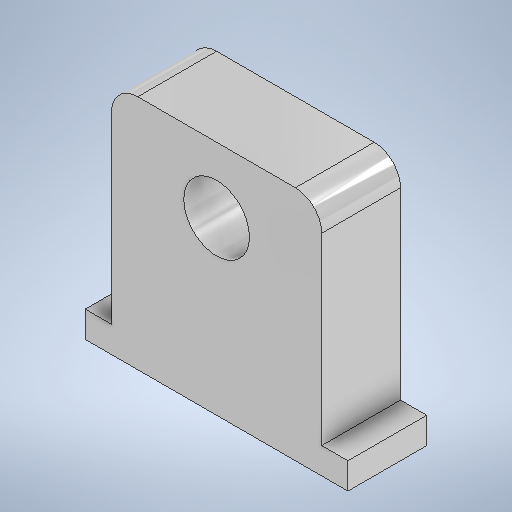
# Autodesk Inventor part: Base
Saved by Autodesk Inventor 2025 (Build 290162000, 162)
## iProperties
Created: 2023-05-05
Part Number: Base
Material: Aluminio 6061
Document SubType Name: Modeling
Designer: Miguel Ángel
Density: 2.69921 g/cm^3
Appearance: Aluminio - Oscuro
Mass: 556 g
Surface Area: 272.311 cm^2
Volume: 205.986 cm^3
Author: Miguel Ángel
Autodesk Inventor part; units mm, degrees
ref_plane "YZ Plane" through (0, 0, 0) normal (1, 0, 0) x (0, 1, 0)
ref_plane "XZ Plane" through (0, 0, 0) normal (0, 1, 0) x (-1, 0, 0)
ref_plane "XY Plane" through (0, 0, 0) normal (0, 0, 1) x (1, 0, 0)
sketch "Boceto1" plane through (0, 0, 0) normal (0, 0, 1) x (1, 0, 0)
  circle A0 centre (0, 0) radius 12.5
  line L0 (0, 25) -> (30, 25)
  line L1 (40, 15) -> (40, -55)
  line L2 (40, -55) -> (50, -55)
  line L3 (50, -55) -> (50, -65)
  line L4 (50, -65) -> (-50, -65)
  line L5 (-50, -65) -> (-50, -55)
  line L6 (-50, -55) -> (-40, -55)
  line L7 (-40, -55) -> (-40, 15)
  line L8 (0, 25) -> (-30, 25)
  arc A1 (-30, 25) -> (-40, 15) centre (-30, 15) ccw
  arc A2 (40, 15) -> (30, 25) centre (30, 15) ccw
  point P0 (40, 25)
  point P1 (-40, 25)
  dimension "d0" = 25
  dimension "d1" = 25
  dimension "d2" = 40
  dimension "d3" = 80
  dimension "d4" = 10
  dimension "d5" = 10
  dimension "d6" = 100
  dimension "d7" = 10
  dimension "d8" = 10
  dimension "d9" = 80
  dimension "d10" = 40
  dimension "d11" = 10
  constraints: 18 end point, 6 point on line, 4 perpendicular, 4 point on circle, 4 tangent, 3 centre point, 2 horizontal, 1 coincident, 1 equal radius
  measures "d0" diameter of A0
  measures "d1" distance of A0.centre L0.start
  measures "d2" distance of L0.start point (40, 25)
  measures "d3" distance of point (40, 25) L1.end
  measures "d4" distance of L1.end L2.end
  measures "d5" distance of L2.end L3.end
  measures "d6" distance of L3.end L4.end
  measures "d7" distance of L4.end L5.end
  measures "d8" distance of L5.end L6.end
  measures "d9" distance of L6.end point (-40, 25)
  measures "d10" distance of L0.start point (-40, 25)
  measures "d11" radius of A1
extrude "Extrusión1" add sketch "Boceto1" along normal blind 30
